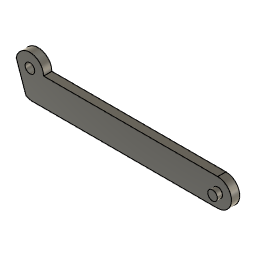
eye_blink_link_up (Autodesk Fusion 360 design; units mm, degrees)
Autodesk Fusion 360 part; units mm, degrees
sketch "Sketch1" plane through (0, 0, 0) normal (0, 0, 1) x (1, 0, 0)
  line L0 (0, 0) -> (27.04, 0)
  line L1 (27.04, 0) -> (27.04, -1.2)
  line L2 (27.04, -1.2) -> (0, -1.2)
  line L3 (0, -1.2) -> (0, 0)
  dimension "d1" = 27.04
  dimension "d2" = 1.2
  constraint horizontal L0
  constraint vertical L1
  constraint horizontal L2
  constraint vertical L3
  constraint coincident L0.start L3.end
  measures "d1" distance of L0.start L0.end
  measures "d2" distance of L0.start L2.end
extrude "Extrude1" add sketch "Sketch1" along normal blind 4
sketch "Sketch2" plane through (0, -1.2, 0) normal (0, -1, 0) x (1, 0, 0)
  line L0 (0, 0) -> (27.04, 0)
  line L1 (27.04, 0) -> (27.04, 4)
  line L2 (27.04, 4) -> (0, 4)
  line L3 (0, 4) -> (0, 0)
  circle A0 centre (27.04, 2) radius 2
  dimension "d5" = 4
  constraint midpoint L1 A0.centre
  measures "d5" diameter of A0
extrude "Extrude2" add sketch "Sketch2" against normal blind 1.2 contours L1 A0 picked at (27.2278, 2.6397)
sketch "Sketch3" plane through (0, -1.2, 0) normal (0, -1, 0) x (1, 0, 0)
  line L0 (0, 0) -> (27.04, 0)
  arc A0 (27.04, 0) -> (27.04, 4) centre (27.04, 2) ccw
  line L1 (27.04, 4) -> (0, 4)
  line L2 (0, 4) -> (0, 0)
  circle A1 centre (27.04, 2) radius 0.7
  dimension "d8" = 1.4
  constraint concentric A0 A1
  measures "d8" diameter of A1
extrude "Extrude3" cut sketch "Sketch3" against normal blind 10 contours A1
sketch "Sketch4" plane through (0, -1.2, 0) normal (0, -1, 0) x (1, 0, 0)
  circle A0 centre (27.04, 2) radius 0.7
  line L0 (0, 0) -> (27.04, 0)
  arc A1 (27.04, 0) -> (27.04, 4) centre (27.04, 2) ccw
  line L1 (27.04, 4) -> (0, 4)
  line L2 (0, 4) -> (0, 0)
  line L3 (0, 0) -> (0, 1.5)
  circle A2 centre (0, 1.5) radius 1.5
  line L4 (-1.0715, 0) -> (5.393, 0) construction
  line L5 (-0.8097, 0) -> (6.2004, 0) construction
  line L6 (25.3, 0) -> (25.3, 4)
  line L7 (25.3, 0) -> (29.5592, 0)
  line L8 (25.3, 4) -> (30.5, 4)
  line L9 (29.04, 0) -> (29.04, 4)
  line L10 (29.04, 4) -> (1.69, 4)
  line L11 (29.04, 4) -> (1.69, 4)
  line L12 (29.04, 4) -> (1.69, 4)
  line L13 (1.69, 4) -> (-0.31, 4)
  circle A3 centre (-0.31, 4) radius 2
  line L14 (1.69, 4) -> (-2.28, 4)
  line L15 (-2.28, 4) -> (-2.28, 4.3451)
  line L16 (1.69, 4) -> (-2.28, 4.3451)
  line L17 (-0.7906, 0) -> (-2.7155, 5.6156)
  line L18 (-0.7906, 0) -> (6.1719, 0) construction
  line L19 (-2.28, 4) -> (29.04, 4)
  dimension "d11" = 1.5
  dimension "d12" = 3
  dimension "d23" = 27.35
  dimension "d24" = 180
  dimension "d25" = 27.35
  dimension "d26" = 2
  dimension "d27" = 4
  dimension "d28" = 3.97
  dimension "d29" = 108.92
  dimension "d30" = 31.32
  constraint coincident L0.start L2.end
  constraint perpendicular L0 L3
  constraint coincident L3.end A2.centre
  constraint horizontal L4
  constraint coincident L0 L4.start
  constraint horizontal L5
  constraint coincident L4 L5.start
  constraint coincident L0 L6.start
  constraint coincident L1 L6.end
  constraint perpendicular L1 L6
  constraint perpendicular L6 L8
  constraint coincident L7 L9.start
  constraint coincident L8 L9.end
  constraint perpendicular L8 L9
  constraint tangent A1 L9
  constraint perpendicular L7 L9
  constraint perpendicular L9 L10
  constraint parallel L1 L13
  constraint coincident L13.end A3.centre
  constraint parallel L1 L14
  constraint coincident A3 L15.end
  constraint perpendicular L14 L15
  constraint horizontal L18
  constraint coincident L4 L17.start
  constraint coincident L15.end L17
  constraint perpendicular L15 L19
  measures "d11" distance of L0.start L3.end
  measures "d12" diameter of A2
  measures "d23" distance of L9.end L10.end
  measures "d24" angle of L11 L12
  measures "d25" distance of L9.end L10.end
  measures "d26" distance of L10.end L13.end
  measures "d27" diameter of A3
  measures "d28" distance of L10.end L14.end
  measures "d29" angle of L17 L18
  measures "d30" distance of L14.end L9.end
extrude "Extrude4" add sketch "Sketch4" against normal blind 1.2 contours L2 L3 A2 A3 L17 | L2 A2 A3 | A2 A3 L17 | A3 L16 | L1 L13 L14 L16 L17 L19 | L2 A2 L13 A3 L14 L17 L19 picked at (-0.163, 2.336)
sketch "Sketch5" plane through (0, -1.2, 0) normal (0, -1, 0) x (1, 0, 0)
  circle A0 centre (27.04, 2) radius 0.7
  line L0 (0, 0) -> (27.04, 0)
  arc A1 (27.04, 0) -> (27.04, 4) centre (27.04, 2) ccw
  line L1 (27.04, 4) -> (1.69, 4)
  arc A2 (1.69, 4) -> (-2.28, 4.3451) centre (-0.31, 4) ccw
  line L2 (-2.28, 4.3451) -> (-0.8912, 0.2935)
  arc A3 (-0.8912, 0.2935) -> (0, 0) centre (0, 1.5) ccw
  circle A4 centre (27.04, 2) radius 0.7
  dimension "d37" = 1.4
  constraint concentric A0 A4
  measures "d37" diameter of A4
sketch "Sketch6" plane through (0, -1.2, 0) normal (0, -1, 0) x (1, 0, 0)
  circle A0 centre (-0.3, 4) radius 0.7
  dimension "d34" = 1.4
  measures "d34" diameter of A0
extrude "Extrude5" cut sketch "Sketch6" against normal blind 6.5
sketch "Sketch7" plane through (0, -1.2, 0) normal (0, -1, 0) x (1, 0, 0)
extrude "Extrude6" add sketch "Sketch5" against normal blind 1.95 contours A0 A4
extrude "Extrude7" add 1 faces at (26.8677, 0.75, 1.935) along direction (0, -1, 0) blind 2.7
